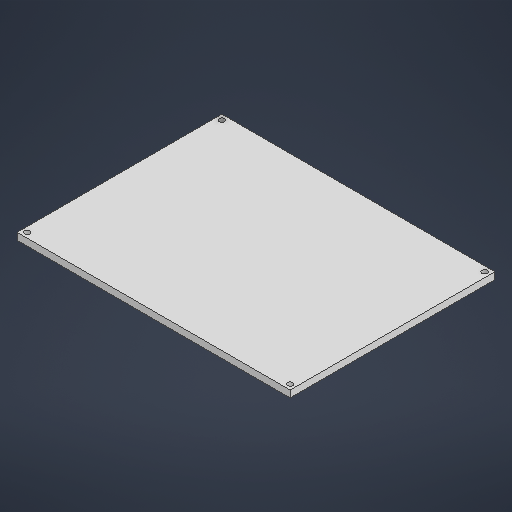
# Autodesk Inventor part: plyta-dolna
Saved by Autodesk Inventor 2026.1 (Build 301233020, 233B)
## iProperties
Created: 2026-02-25
Part Number: plyta-dolna
Material: Generic
Document SubType Name: Modeling
Designer: Jan
Density: 1 g/cm^3
Appearance: Default
Author: Jan
Autodesk Inventor part; units mm, degrees
ref_plane "YZ Plane" through (0, 0, 0) normal (1, 0, 0) x (0, 1, 0)
ref_plane "XZ Plane" through (0, 0, 0) normal (0, 1, 0) x (-1, 0, 0)
ref_plane "XY Plane" through (0, 0, 0) normal (0, 0, 1) x (1, 0, 0)
sketch "Sketch1" plane through (0, 0, 0) normal (0, 1, 0) x (-1, 0, 0)
  line L0 (0, 0) -> (-160, 0)
  line L1 (-160, 0) -> (-160, -120)
  line L2 (-160, -120) -> (0, -120)
  line L3 (0, -120) -> (0, 0)
  dimension "d0" = 160
  dimension "d1" = 120
  constraints: 8 end point, 2 parallel, 1 horizontal, 1 perpendicular
  measures "d0" distance of L2.end L1.end
  measures "d1" distance of L1.end L0.end
extrude "Extrusion1" add sketch "Sketch1" along normal blind 4
sketch "Sketch2" plane through (0, 0, 0) normal (0, -1, 0) x (1, 0, 0)
  line L0 (157, -3) -> (3, -3) construction
  line L1 (3, -3) -> (3, -117) construction
  line L2 (3, -117) -> (157, -117) construction
  line L3 (157, -117) -> (157, -3) construction
  line L4 (0, 0) -> (160, 0) construction
  line L5 (160, -120) -> (0, -120) construction
  line L6 (160, 0) -> (160, -120) construction
  line L7 (0, -120) -> (0, 0) construction
  circle A0 centre (157, -3) radius 1 construction
  circle A1 centre (157, -117) radius 1 construction
  circle A2 centre (3, -117) radius 1 construction
  circle A3 centre (3, -3) radius 1 construction
  dimension "d4" = 3
  dimension "d5" = 3
  dimension "d6" = 3
  dimension "d7" = 3
  dimension "d8" = 2
  dimension "d9" = 2
  dimension "d10" = 2
  dimension "d11" = 2
  constraints: 8 end point, 4 centre point, 4 coincident, 2 parallel, 1 horizontal, 1 perpendicular
  measures "d4" distance between parallel lines of L4 L0
  measures "d5" distance between parallel lines of L5 L2
  measures "d6" distance between parallel lines of L6 L3
  measures "d7" distance between parallel lines of L1 L7
  measures "d8" diameter of A0
  measures "d9" diameter of A1
  measures "d10" diameter of A2
  measures "d11" diameter of A3
hole "Hole1" at (3, 0, -3) at (3, 0, -117) at (157, 0, -117) at (157, 0, -3) direction (0, 1, 0) diameter 3.2 depth 7.2 tip angle 118
chamfer "Chamfer1" distance 0.3 angle 45 4 edges at (157, 0, -115.4) (3, 0, -115.4) (157, 0, -1.4) (3, 0, -1.4)
equation "\"d4\" = d5"
equation "\"d6\" = d5"
equation "\"d7\" = d5"
body "Solid1"
